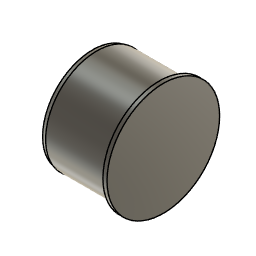
Stopfen DN50 v1 (Autodesk Fusion 360 design; units mm, degrees)
Autodesk Fusion 360 part; units mm, degrees
sketch "Skizze1" plane through (0, 0, 0) normal (0, 0, 1) x (1, 0, 0)
  line L0 (0, 0) -> (0, 27.5)
  line L1 (0, 27.5) -> (-2, 27.5)
  line L2 (-2, 27.5) -> (-2, 25)
  line L3 (-2, 25) -> (-32.5, 25)
  line L4 (-32.5, 25) -> (-34.5, 24.4641)
  line L5 (-34.5, 24.4641) -> (-34.5, 23)
  line L6 (-34.5, 23) -> (-2, 23)
  line L7 (-2, 23) -> (-2, 0)
  line L8 (-2, 0) -> (0, 0)
  dimension "d2" = 27.5
  dimension "d3" = 32.5
  dimension "d4" = 2
  dimension "d5" = 23
  dimension "d6" = 25
  dimension "d7" = 15
  dimension "d8" = 2
  constraint coincident L0.start L8.end
  constraint vertical L0
  constraint perpendicular L0 L1
  constraint perpendicular L1 L2
  constraint perpendicular L2 L3
  constraint perpendicular L3 L5
  constraint perpendicular L5 L6
  constraint perpendicular L6 L7
  constraint perpendicular L0 L8
  constraint collinear L2 L7
  measures "d2" distance of L0.start L0.end
  measures "d3" distance of L5.end L6.end
  measures "d4" distance of L0.end L1.end
  measures "d5" distance of L6.end L7.end
  measures "d6" distance of L3 L8
  measures "d7" angle of L3 L4
  measures "d8" distance of L3.end L5
revolve "Drehen1" add sketch "Skizze1" angle 360 about axis through (1.75, 0, 0) along (1, 0, 0)
equation "d2 = ( 55 / 2 ) * 1 mm"
equation "d5 = ( 46 / 2 ) * 1 mm"
equation "d6 = ( 50 / 2 ) * 1 mm"
